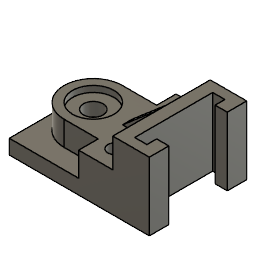
Part1CAD (Autodesk Fusion 360 design; units mm, degrees)
part number: 2026-04-19-09-28-07-422
Autodesk Fusion 360 part; units mm, degrees
note: some values were not read from the file. Chosen so that the rebuilt part matches the saved one: which face or edge a step refers to. Set by a fixed rule: which sketch regions a step uses.
sketch "Sketch1" plane through (0, 0, 0) normal (0, 1, 0) x (1, 0, 0)
  line L0 (0, 0) -> (115, 0)
  line L1 (115, 0) -> (115, -80)
  line L2 (115, -80) -> (0, -80)
  line L3 (0, -80) -> (0, 0)
  line L4 (115, -40) -> (0, -40)
  line L5 (115, -40) -> (115, -16)
  line L6 (115, -16) -> (115, 0)
  line L7 (115, -40) -> (115, -41)
  line L8 (115, -40) -> (115, -64)
  line L9 (115, -64) -> (115, -80)
  line L10 (115, -80) -> (85, -80)
  line L11 (115, 0) -> (85, 0)
  line L12 (85, 0) -> (85, -80)
  line L13 (115, -40) -> (115, -16)
  line L14 (115, -16) -> (105, -16)
  line L15 (105, -16) -> (105, -8)
  line L16 (105, -8) -> (95, -8)
  line L17 (115, -40) -> (115, -41)
  line L18 (115, -40) -> (115, -64)
  line L19 (115, -64) -> (105, -64)
  line L20 (105, -64) -> (105, -72)
  line L21 (105, -72) -> (95, -72)
  line L22 (95, -72) -> (95, -8)
  line L23 (85, -40) -> (57, -40)
  line L24 (57, -40) -> (85, -40)
  line L25 (85, -40) -> (85, -36)
  line L26 (85, -36) -> (57, -36)
  line L27 (57, -36) -> (57, -40)
  line L28 (57, -40) -> (85, -40)
  line L29 (85, -40) -> (85, -44)
  line L30 (85, -44) -> (57, -44)
  line L31 (57, -44) -> (57, -40)
  line L32 (85, -80) -> (71, -80)
  line L33 (71, -80) -> (71, -64)
  line L34 (71, -64) -> (85, -64)
  line L35 (85, -64) -> (85, -80)
  line L36 (85, 0) -> (71, 0)
  line L37 (71, 0) -> (71, -16)
  line L38 (71, -16) -> (85, -16)
  line L39 (85, -16) -> (85, 0)
  circle A0 centre (71, -16) radius 6
  circle A1 centre (71, -64) radius 6
  line L40 (57, -40) -> (29, -40)
  circle A2 centre (29, -40) radius 24
  line L41 (57, -80) -> (57, -64)
  line L42 (57, -64) -> (29, -64)
  line L43 (57, 0) -> (57, -16)
  line L44 (57, -16) -> (29, -16)
  dimension "d1" = 115
  dimension "d2" = 80
  dimension "d25" = 28
  dimension "d26" = 28
  dimension "d27" = 4
  dimension "d28" = 28
  dimension "d29" = 4
  dimension "d30" = 14
  dimension "d31" = 16
  dimension "d32" = 14
  dimension "d33" = 16
  dimension "d34" = 12
  dimension "d35" = 12
  dimension "d36" = 28
  dimension "d37" = 48
  dimension "d42" = 16
  dimension "d43" = 16
  constraint horizontal L0
  constraint vertical L1
  constraint horizontal L2
  constraint vertical L3
  constraint coincident L0.start L3.end
  constraint midpoint L1 L4.start
  constraint midpoint L3 L4.end
  constraint perpendicular L4 L5
  constraint parallel L1 L6
  constraint coincident L1 L7.end
  constraint perpendicular L4 L8
  constraint vertical L9
  constraint perpendicular L1 L10
  constraint perpendicular L6 L11
  constraint perpendicular L4 L13
  constraint perpendicular L1 L14
  constraint perpendicular L14 L15
  constraint perpendicular L15 L16
  constraint perpendicular L4 L18
  constraint perpendicular L1 L19
  constraint perpendicular L19 L20
  constraint perpendicular L20 L21
  constraint midpoint L12 L23.start
  constraint perpendicular L12 L23
  constraint horizontal L24
  constraint vertical L25
  constraint horizontal L26
  constraint vertical L27
  constraint horizontal L28
  constraint vertical L29
  constraint horizontal L30
  constraint vertical L31
  constraint horizontal L32
  constraint vertical L33
  constraint horizontal L34
  constraint vertical L35
  constraint horizontal L36
  constraint vertical L37
  constraint horizontal L38
  constraint vertical L39
  constraint coincident L37.end L38.start
  constraint coincident L33.end L34.start
  constraint horizontal L40
  constraint coincident L40.end A2.centre
  constraint coincident L2 L41.start
  constraint perpendicular L2 L41
  constraint coincident A2 L42.end
  constraint tangent A2 L42
  constraint coincident L0 L43.start
  constraint perpendicular L0 L43
  constraint coincident A2 L44.end
  constraint tangent A2 L44
  constraint perpendicular L43 L44
  measures "d1" distance of L0.start L0.end
  measures "d2" distance of L0.start L2.end
  measures "d25" distance of L23.start L23.end
  measures "d26" distance of L23.end L23.start
  measures "d27" distance of L23.end L26.end
  measures "d28" distance of L23.end L23.start
  measures "d29" distance of L23.end L30.end
  measures "d30" distance of L10.end L32.end
  measures "d31" distance of L10.end L34.end
  measures "d32" distance of L11.end L36.end
  measures "d33" distance of L11.end L38.end
  measures "d34" diameter of A0
  measures "d35" diameter of A1
  measures "d36" distance of L23.end L40.end
  measures "d37" diameter of A2
  measures "d42" distance of L41.start L41.end
  measures "d43" distance of L43.start L43.end
extrude "Extrude1" add sketch "Sketch1" along normal blind 56 contours L0 L1 L4 L6 L11 L12 L14 L15 L16 L22 L25 L39 | L1 L2 L4 L9 L10 L12 L19 L20 L21 L22 L29 L35
extrude "Extrude2" add sketch "Sketch1" along normal blind 56 contours L4 L12 L23 L24 L25 L26 L27 L28 | L4 L12 L23 L24 L28 L29 L30 L31
extrude "Extrude3" cut 1 faces at (91.6667, 56, 38.6667) along direction (0, -1, 0) blind 60
extrude "Extrude4" add sketch "Sketch1" along normal blind 56 contours L0 L1 L4 L6 L11 L12 L14 L15 L16 L22 L25 L39 | L1 L2 L4 L9 L10 L12 L19 L20 L21 L22 L29 L35
extrude "Extrude5" add sketch "Sketch1" along normal blind 32 contours L0 L4 L12 L26 L27 L37 L38 A0 L40 A2 L43 L44 | L0 L12 L36 L37 L38 L39 A0 | L4 L40 A2 | L4 L40 A2 | L2 L4 L12 L30 L31 L33 L34 A1 L40 A2 L41 L42 | L2 L12 L32 L33 L34 L35 A1 | L4 L12 L23 L24 L25 L26 L27 L28 | L4 L12 L23 L24 L28 L29 L30 L31
extrude "Extrude6" add sketch "Sketch1" along normal blind 12 contours L0 L3 L4 A2 L43 L44 | L2 L3 L4 A2 L41 L42
sketch "Sketch2" plane through (0, 32, 0) normal (0, 1, 0) x (-1, 0, 0)
  circle A0 centre (-71, 64) radius 6
  circle A1 centre (-71, 16) radius 6
  line L0 (-57, 0) -> (-57, 16)
  line L1 (-57, 16) -> (-29, 16)
  arc A2 (-29, 16) -> (-29, 64) centre (-29, 40) ccw
  line L2 (-29, 64) -> (-57, 64)
  line L3 (-57, 64) -> (-57, 80)
  line L4 (-57, 80) -> (-85, 80)
  line L5 (-85, 80) -> (-85, 0)
  line L6 (-85, 0) -> (-57, 0)
  line L7 (-85, 40) -> (-57, 40)
  line L8 (-57, 40) -> (-85, 40)
  line L9 (-85, 40) -> (-85, 36)
  line L10 (-85, 36) -> (-57, 36)
  line L11 (-57, 36) -> (-57, 40)
  line L12 (-57, 40) -> (-85, 40)
  line L13 (-85, 40) -> (-85, 44)
  line L14 (-85, 44) -> (-57, 44)
  line L15 (-57, 44) -> (-57, 40)
  dimension "d52" = 28
  dimension "d53" = 28
  dimension "d54" = 4
  dimension "d55" = 4
  constraint midpoint L5 L7.start
  constraint perpendicular L5 L7
  constraint horizontal L8
  constraint vertical L9
  constraint horizontal L10
  constraint vertical L11
  constraint horizontal L12
  constraint vertical L13
  constraint horizontal L14
  constraint vertical L15
  measures "d52" distance of L7.start L7.end
  measures "d53" distance of L7.end L7.start
  measures "d54" distance of L7.end L10.end
  measures "d55" distance of L7.end L14.end
sketch "Sketch3" plane through (85, 0, 0) normal (-1, 0, 0) x (0, 0, 1)
  line L0 (0, 32) -> (80, 32)
  line L1 (80, 32) -> (80, 56)
  line L2 (80, 56) -> (0, 56)
  line L3 (0, 56) -> (0, 32)
  line L4 (40, 56) -> (40, 32)
  line L5 (40, 56) -> (36, 56)
  line L6 (40, 56) -> (44, 56)
  line L7 (36, 56) -> (36, 32)
  line L8 (44, 56) -> (44, 32)
  dimension "d56" = 4
  dimension "d57" = 4
  constraint midpoint L2 L4.start
  constraint midpoint L0 L4.end
  constraint perpendicular L4 L5
  constraint perpendicular L4 L6
  constraint coincident L0 L7.end
  constraint perpendicular L0 L7
  constraint coincident L0 L8.end
  constraint perpendicular L0 L8
  measures "d56" distance of L4.start L5.end
  measures "d57" distance of L4.start L6.end
sketch "Sketch4" plane through (85, 0, 0) normal (-1, 0, 0) x (0, 0, 1)
sketch "Sketch5" plane through (0, 32, 0) normal (0, 1, 0) x (-1, 0, 0)
sketch "Sketch6" plane through (0, 32, 0) normal (0, 1, 0) x (-1, 0, 0)
  line L0 (-57, 64) -> (-29, 64)
  line L1 (-29, 64) -> (-29, 16)
  circle A0 centre (-29, 40) radius 17
  circle A1 centre (-29, 40) radius 8
  dimension "d58" = 28
  dimension "d71" = 34
  dimension "d72" = 16
  constraint horizontal L0
  constraint perpendicular L0 L1
  constraint midpoint L1 A0.centre
  constraint concentric A0 A1
  measures "d58" distance of L0.start L0.end
  measures "d71" diameter of A0
  measures "d72" diameter of A1
hole "Hole1" at (29, 32, 40) direction (0, -1, 0) diameter 16 depth 5 tip angle 180 counterbore diameter 34 counterbore depth 5
sketch "Sketch7" plane through (0, 0, 0) normal (0, 0, 1) x (1, 0, 0)
sketch "Sketch8" plane through (0, 0, 80) normal (0, 0, 1) x (1, 0, 0)
  line L0 (0, 0) -> (115, 0)
  line L1 (115, 0) -> (115, 56)
  line L2 (115, 56) -> (85, 56)
  line L3 (85, 56) -> (85, 32)
  line L4 (85, 32) -> (57, 32)
  line L5 (57, 32) -> (57, 12)
  line L6 (57, 12) -> (0, 12)
  line L7 (0, 12) -> (0, 0)
  line L8 (85, 32) -> (57, 32)
  line L9 (57, 32) -> (85, 56)
  dimension "d64" = 28
  constraint coincident L3.end L4.start
  constraint perpendicular L3 L8
  constraint coincident L2.end L3.start
  measures "d64" distance of L3.end L4.end
sketch "Sketch9" plane through (0, 32, 0) normal (0, 1, 0) x (-1, 0, 0)
  circle A0 centre (-29, 40) radius 17
  circle A1 centre (-71, 64) radius 6
  circle A2 centre (-71, 16) radius 6
  line L0 (-57, 0) -> (-57, 16)
  line L1 (-57, 16) -> (-29, 16)
  arc A3 (-29, 16) -> (-29, 64) centre (-29, 40) ccw
  line L2 (-29, 64) -> (-57, 64)
  line L3 (-57, 64) -> (-57, 80)
  line L4 (-57, 80) -> (-85, 80)
  line L5 (-85, 80) -> (-85, 0)
  line L6 (-85, 0) -> (-57, 0)
extrude "Extrude7" add sketch "Sketch3" against normal blind 1 contours L0 L2 L4 L6 L8
sketch "Sketch10" plane through (0, 0, 44) normal (0, 0, 1) x (1, 0, 0)
  line L0 (85, 32) -> (85, 56)
  line L1 (85, 56) -> (83, 56)
  line L2 (83, 56) -> (83, 32)
  line L3 (83, 32) -> (85, 32)
  line L4 (85, 56) -> (57, 32)
  line L5 (57, 32) -> (85, 32)
  line L6 (85, 32) -> (85, 56)
  constraint coincident L0.end L1.start
  constraint coincident L0.start L3.end
extrude "Extrude8" add sketch "Sketch10" against normal blind 8 contours L0 L2 L3 L4 L5 L6 | L2 L4 L5
extrude "Extrude9" add 1 faces at (38.6535, 27, 39.0485) along direction (0, 1, 0) blind 5
sketch "Sketch11" plane through (0, 32, 0) normal (0, 1, 0) x (-1, 0, 0)
hole "Hole2" at (29, 32, 40) direction (0, -1, 0) diameter 16 depth 16 tip angle 180 counterbore diameter 34 counterbore depth 5
